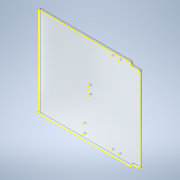
# Autodesk Inventor part: BottomAcrylicSheet
Saved by Autodesk Inventor 2021 (Build 250183000, 183)
## iProperties
Created: 2020-07-16
Part Number: BottomAcrylicSheet
Material: Generic
Document SubType Name: Modeling
Designer: CASE-SMALL2
Density: 1 g/cm^3
Appearance: Default
Author: CASE-SMALL2
Autodesk Inventor part; units mm, degrees
ref_plane "YZ Plane" through (0, 0, 0) normal (1, 0, 0) x (0, 1, 0)
ref_plane "XZ Plane" through (0, 0, 0) normal (0, 1, 0) x (-1, 0, 0)
ref_plane "XY Plane" through (0, 0, 0) normal (0, 0, 1) x (1, 0, 0)
sketch "Sketch1" plane through (0, 0, 0) normal (0, 0, 1) x (1, 0, 0)
  line L0 (-112.5, -100) -> (112.5, -100)
  line L1 (112.5, -100) -> (112.5, 100)
  line L2 (112.5, 100) -> (-112.5, 100)
  line L3 (-112.5, 100) -> (-112.5, -100)
  line L4 (-112.5, -100) -> (112.5, 100) construction
  line L5 (112.5, -100) -> (-112.5, 100) construction
  point P0 (0, 0)
  dimension "d0" = 225
  dimension "d1" = 200
  constraints: 12 end point, 2 midpoint, 2 parallel, 1 horizontal, 1 perpendicular
  measures "d0" distance of L1.end L2.end
  measures "d1" distance of L0.end L1.end
extrude "Extrusion1" add sketch "Sketch1" along normal blind 5
sketch "Sketch2" plane through (0, 0, 5) normal (0, 0, 1) x (1, 0, 0)
  point P0 (0, 0)
sketch "Sketch3" plane through (0, 0, 5) normal (0, 0, 1) x (1, 0, 0)
  circle A0 centre (65.5, -90) radius 1.75
  circle A1 centre (49.5, -90) radius 1.75
  circle A2 centre (65.5, 90) radius 1.75
  circle A3 centre (49.5, 90) radius 1.75
  line L0 (-112.5, -100) -> (112.5, -100) projected
  line L1 (112.5, 100) -> (-112.5, 100) projected
  line L2 (112.5, -100) -> (112.5, 100) projected
  point P0 (0, 0)
  dimension "d4" = 3.5
  dimension "d5" = 3.5
  dimension "d6" = 3.5
  dimension "d7" = 3.5
  dimension "d8" = 16
  dimension "d9" = 16
  dimension "d10" = 10
  dimension "d11" = 10
  dimension "d12" = 47
  dimension "d13" = 47
  constraints: 4 centre point
  measures "d4" diameter of A0
  measures "d5" diameter of A1
  measures "d6" diameter of A2
  measures "d7" diameter of A3
  measures "d8" distance of A1.centre A0.centre
  measures "d9" distance of A3.centre A2.centre
  measures "d10" distance from line of L0 A0.centre
  measures "d11" distance from line of L1 A2.centre
  measures "d12" distance from line of L2 A0.centre
  measures "d13" distance from line of L2 A2.centre
extrude "Extrusion2" cut sketch "Sketch3" against normal through all
sketch "Sketch4" plane through (0, 0, 5) normal (0, 0, 1) x (1, 0, 0)
  circle A0 centre (-12.5, -90) radius 1.75
  circle A1 centre (-12.5, -70) radius 1.75
  circle A2 centre (49.5, -90) radius 1.75 projected
  line L0 (-112.5, -100) -> (112.5, -100) projected
  line L1 (-112.5, 100) -> (-112.5, -100) projected
  point P0 (0, 0)
  point P1 (-110.5, -100)
  point P2 (110.5, -100)
  point P3 (-112.5, 98)
  point P4 (-112.5, -98)
  dimension "d18" = 3.5
  dimension "d19" = 3.5
  dimension "d26" = 3.5
  dimension "d27" = 10
  dimension "d28" = 20
  dimension "d29" = 100
  dimension "d30" = 100
  constraints: 2 centre point
  measures "d18" diameter of A2
  measures "d19" diameter of A0
  measures "d26" diameter of A1
  measures "d27" distance from line of L0 A0.centre
  measures "d28" distance of A0.centre A1.centre
  measures "d29" distance from line of L1 A1.centre
  measures "d30" distance from line of L1 A0.centre
extrude "Extrusion3" cut sketch "Sketch4" against normal through all contours A0 | A1
sketch "Sketch5" plane through (0, 0, 5) normal (0, 0, 1) x (1, 0, 0)
  line L0 (0, -140.5799) -> (0, 140.5799) construction
  circle A0 centre (0, -9) radius 1.75
  circle A1 centre (0, 9) radius 1.75
  point P0 (0, 0)
  dimension "d31" = 3.5
  dimension "d32" = 3.5
  dimension "d33" = 9
  dimension "d34" = 9
  constraints: 2 centre point, 2 point on line
  measures "d31" diameter of A0
  measures "d32" diameter of A1
  measures "d33" distance of point (0, 0) A0.centre
  measures "d34" distance of point (0, 0) A1.centre
extrude "Extrusion4" cut sketch "Sketch5" against normal through all
sketch "Sketch7" plane through (0, 0, 5) normal (0, 0, 1) x (1, 0, 0)
  line L0 (112.5, -100) -> (112.5, 100) construction
  line L1 (112.5, -100) -> (92.5, -100)
  line L2 (92.5, -100) -> (92.5, -94)
  line L3 (92.5, -94) -> (112.5, -94)
  line L4 (112.5, -94) -> (112.5, -100)
  line L5 (131.6327, 0) -> (-168.572, 0) construction
  line L6 (-112.5, -100) -> (112.5, -100) construction
  line L7 (112.5, 100) -> (-112.5, 100) projected
  line L8 (112.5, 100) -> (92.5, 100)
  line L9 (92.5, 100) -> (92.5, 94)
  line L10 (92.5, 94) -> (112.5, 94)
  line L11 (112.5, 94) -> (112.5, 100)
  point P0 (0, 0)
  dimension "d37" = 20
  dimension "d38" = 6
  dimension "d39" = 100
  dimension "d40" = 200
  constraints: 18 end point, 3 symmetric about line, 2 horizontal, 2 parallel, 1 perpendicular
  measures "d37" distance of L2.end L3.end
  measures "d38" distance between parallel lines of L3 L1
  measures "d39" distance between parallel lines of L5 L6
  measures "d40" distance between parallel lines of L7 L6
extrude "Extrusion5" cut sketch "Sketch7" against normal through all
fillet "Fillet2" radius 2 8 edges at (112.5, -94, 2.5) (92.5, -94, 2.5) (92.5, -100, 2.5) (112.5, 94, 2.5) (92.5, 94, 2.5) (92.5, 100, 2.5) (-112.5, 100, 2.5) (-112.5, -100, 2.5)
sketch "Sketch8" plane through (0, 0, 5) normal (0, 0, 1) x (1, 0, 0)
  arc A0 (-112.5, -98) -> (-110.5, -100) centre (-110.5, -98) ccw projected
  line L0 (-110.5, -100) -> (90.5, -100) projected
  arc A1 (90.5, -100) -> (92.5, -98) centre (90.5, -98) ccw projected
  line L1 (92.5, -98) -> (92.5, -96) projected
  arc A2 (94.5, -94) -> (92.5, -96) centre (94.5, -96) ccw projected
  line L2 (94.5, -94) -> (110.5, -94) projected
  arc A3 (110.5, -94) -> (112.5, -92) centre (110.5, -92) ccw projected
  line L3 (112.5, -92) -> (112.5, 92) projected
  arc A4 (112.5, 92) -> (110.5, 94) centre (110.5, 92) ccw projected
  line L4 (110.5, 94) -> (94.5, 94) projected
  arc A5 (92.5, 96) -> (94.5, 94) centre (94.5, 96) ccw projected
  line L5 (92.5, 96) -> (92.5, 98) projected
  arc A6 (92.5, 98) -> (90.5, 100) centre (90.5, 98) ccw projected
  line L6 (90.5, 100) -> (-110.5, 100) projected
  arc A7 (-110.5, 100) -> (-112.5, 98) centre (-110.5, 98) ccw projected
  line L7 (-112.5, 98) -> (-112.5, -98) projected
  circle A8 centre (65.5, -90) radius 1.75 projected
  circle A9 centre (49.5, 90) radius 1.75 projected
  circle A10 centre (49.5, -90) radius 1.75 projected
  circle A11 centre (65.5, 90) radius 1.75 projected
  circle A12 centre (-12.5, -70) radius 1.75 projected
  circle A13 centre (-12.5, -90) radius 1.75 projected
  circle A14 centre (0, -9) radius 1.75 projected
  circle A15 centre (0, 9) radius 1.75 projected
  point P0 (0, 0)
equation "\"d5\" = d4"
equation "\"d6\" = d4"
equation "\"d7\" = d4"
equation "\"d11\" = d10"
equation "\"d13\" = d12"
equation "\"d19\" = d18"
equation "\"d26\" = d19"
equation "\"d30\" = d29"
equation "\"d32\" = d31"
equation "\"d34\" = d33"
equation "\"d39\" = 0.5 * d40"
body "Solid1"
